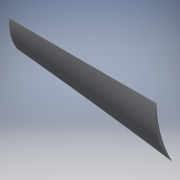
# Autodesk Inventor part: test_front_element_1
Saved by Autodesk Inventor 2018.1 (Build 221171000, 171)
## iProperties
Created: 2017-10-30
Part Number: test_front_element_1
Material: 一般
Document SubType Name: Modeling
Designer: ku_sk
Density: 1 g/cm^3
Appearance: 既定
Author: ku_sk
Autodesk Inventor part; units mm, degrees
ref_plane "XZ Plane" through (0, 0, 0) normal (0, 1, 0) x (-1, 0, 0)
ref_plane "作業平面1" through (150, 0, 0) normal (1, 0, 0) x (0, 1, 0)
ref_plane "作業平面2" through (325, 0, 0) normal (1, 0, 0) x (0, 1, 0)
sketch "スケッチ2" plane through (0, 0, 0) normal (1, 0, 0) x (0, 1, 0)
  arc A0 (0.1333, -0.9307) -> (18.4066, -69.1273) centre (297.0345, 42.0773) ccw
  arc A1 (-0.0654, -0.9385) -> (18.2305, -69.2199) centre (109.7, -8.1189) ccw
  line L0 (0, -93.2911) -> (0, 64.6387) projected
  line L1 (0, 0) -> (18.7564, -70)
  arc A2 (18.2305, -69.2199) -> (18.4066, -69.1273) centre (18.3137, -69.1644) ccw
  arc A3 (0.1333, -0.9307) -> (-0.0654, -0.9385) centre (0.0344, -0.945) ccw
  dimension "d6" = 70
  dimension "d8" = 15
  dimension "d9" = 0.1
  dimension "d10" = 0.1
  dimension "d31" = 300
  dimension "d32" = 110
  constraints: 12 point on circle, 4 centre point, 4 tangent, 2 end point, 1 coincident
  measures "d6" vertical distance of L1.end L1.start
  measures "d8" angle of L0 L1
  measures "d9" radius of A2
  measures "d10" radius of A3
  measures "d31" radius of A0
  measures "d32" radius of A1
sketch "スケッチ3" plane through (150, 0, 0) normal (1, 0, 0) x (0, 1, 0)
  line L0 (0, 0) -> (20.7781, -90)
  arc A0 (0.1096, -1.4627) -> (20.2354, -88.6373) centre (299.2155, 21.6808) ccw
  arc A1 (-0.09, -1.4648) -> (20.0552, -88.7229) centre (159.6525, -10.5398) ccw
  line L1 (0, -112.5294) -> (0, 44.0492) projected
  arc A2 (20.0552, -88.7229) -> (20.2354, -88.6373) centre (20.1424, -88.674) ccw
  arc A3 (0.1096, -1.4627) -> (-0.09, -1.4648) centre (0.0099, -1.4705) ccw
  dimension "d11" = 13
  dimension "d12" = 90
  dimension "d13" = 0.1
  dimension "d29" = 300
  dimension "d30" = 160
  constraints: 12 point on circle, 4 centre point, 4 tangent, 2 end point, 1 equal radius
  measures "d11" angle of L1 L0
  measures "d12" vertical distance of L0.start L0.end
  measures "d13" radius of A2
  measures "d29" radius of A0
  measures "d30" radius of A1
sketch "スケッチ4" plane through (325, 0, 0) normal (1, 0, 0) x (0, 1, 0)
  line L0 (0, 0) -> (34.8334, -130)
  arc A0 (0.0359, -0.9645) -> (34.3822, -129.1468) centre (299.8103, 10.6671) ccw
  arc A1 (-0.1627, -0.9519) -> (34.2166, -129.257) centre (157.6313, -27.4296) ccw
  line L1 (0, -161.7253) -> (0, 39.3992) projected
  arc A2 (34.2166, -129.257) -> (34.3822, -129.1468) centre (34.2937, -129.1934) ccw
  arc A3 (0.0359, -0.9645) -> (-0.1627, -0.9519) centre (-0.0641, -0.9684) ccw
  dimension "d18" = 15
  dimension "d19" = 130
  dimension "d20" = 0.1
  dimension "d27" = 300
  dimension "d28" = 160
  constraints: 12 point on circle, 4 centre point, 4 tangent, 2 end point, 1 equal radius
  measures "d18" angle of L1 L0
  measures "d19" vertical distance of L0.start L0.end
  measures "d20" radius of A2
  measures "d27" radius of A0
  measures "d28" radius of A1
loft "ロフト2" add profiles "スケッチ2", "スケッチ3", "スケッチ4"
